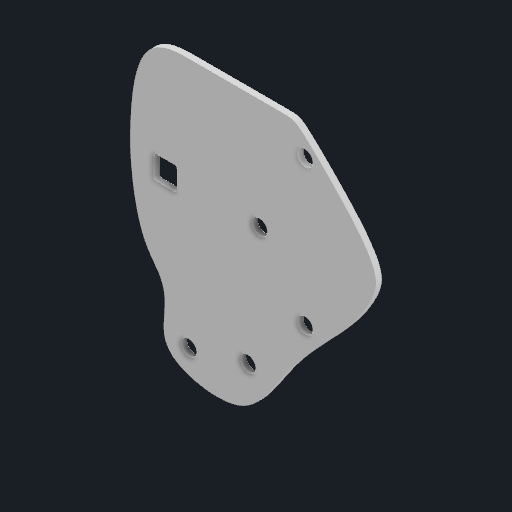
# Autodesk Inventor part: tracking-wheet-outer-mount-v2
Saved by Autodesk Inventor 2023.2 (Build 272271000, 271)
## iProperties
Created: 2023-04-12
Part Number: tracking-wheet-outer-mount-v2
Material: Generic
Document SubType Name: Modeling
Designer: Liam
Density: 1 g/cm^3
Appearance: Default
Author: Liam
Autodesk Inventor part; units mm, degrees
ref_plane "YZ Plane" through (0, 0, 0) normal (1, 0, 0) x (0, 1, 0)
ref_plane "XZ Plane" through (0, 0, 0) normal (0, 1, 0) x (-1, 0, 0)
ref_plane "XY Plane" through (0, 0, 0) normal (0, 0, 1) x (1, 0, 0)
sketch "Sketch1" plane through (0, 0, 0) normal (0, 0, 1) x (1, 0, 0)
  circle A0 centre (13.9823, 30.134) radius 2.0955 projected
  circle A1 centre (13.9823, -8.8165) radius 2.0955 projected
  circle A2 centre (-1.3811, -25.4474) radius 2.0955 projected
  circle A3 centre (-17.2724, -29.6635) radius 2.0955 projected
  line L0 (-20.518, 10.4175) -> (-20.518, 5.3883)
  line L1 (-21.153, 4.7533) -> (-26.1822, 4.7533)
  line L2 (-26.8172, 5.3883) -> (-26.8172, 10.4175)
  line L3 (-26.1822, 11.0525) -> (-21.153, 11.0525)
  arc A4 (-20.518, 10.4175) -> (-21.153, 11.0525) centre (-21.153, 10.4175) ccw
  arc A5 (-21.153, 4.7533) -> (-20.518, 5.3883) centre (-21.153, 5.3883) ccw
  arc A6 (-26.8172, 5.3883) -> (-26.1822, 4.7533) centre (-26.1822, 5.3883) ccw
  arc A7 (-26.1822, 11.0525) -> (-26.8172, 10.4175) centre (-26.1822, 10.4175) ccw
  line L4 (-23.6676, 7.9029) -> (-23.6676, 4.7533) construction
  line L5 (-23.6676, 7.9029) -> (-20.518, 7.9029) construction
  circle A8 centre (1.7324, 7.9029) radius 2.0955
  spline S0 degree 4 poles (-33.0614, 10.6587) (-33.0614, 4.3619) (-30.7457, -10.912) (-26.1565, -14.0262) (-21.9406, -21.3181) (-26.8507, -33.1) (-14.4545, -37.7063) (-3.2273, -37.7063) (3.1129, -31.759) (9.04, -21.3181) (16.0778, -13.5219) (22.0281, -7.3551) (28.8094, -0.0648) (33.0614, 7.9099) (33.0614, 10.6587) knots -12 -12 -12 -12 -12 -11 -10 -9 -8 -7 -6 -5 -4 -3 -2 -1 -1 -1 -1 -1 projected
  spline S1 degree 4 poles (33.0614, 10.6587) (33.0614, 15.0888) (24.5573, 25.0103) (12.2936, 37.1336) (10.8364, 37.7063) (6.7243, 37.7063) (3.0914, 37.7063) (-3.2273, 37.7063) (-7.0886, 37.7063) (-21.8204, 37.7063) (-24.0886, 37.7063) (-33.0614, 31.906) (-33.0614, 10.6587) knots -10 -10 -10 -10 -10 -9 -8 -7 -6 -5 -4 -3 -2 -1 -1 -1 -1 -1 projected
  point P0 (0, 0)
  point P1 (-20.518, 11.0525)
  point P2 (-20.518, 4.7533)
  dimension "d0" = 6.2992
  dimension "d1" = 0.635
  dimension "d2" = 3.1496
  dimension "d3" = 3.1496
  dimension "d4" = 4.191
  dimension "d5" = 0
  dimension "d6" = 25.4
  constraints: 12 end point, 8 point on circle, 8 tangent, 5 centre point, 4 point on line, 3 equal radius, 3 perpendicular, 2 midpoint, 1 horizontal, 1 vertical, 1 other
  measures "d0" distance of point (-20.518, 11.052) point (-20.518, 4.753)
  measures "d1" radius of A4
  measures "d2" distance of L4.start L5.end
  measures "d3" distance of L4.start L4.end
  measures "d4" diameter of A8
  measures "d5" vertical distance of L4.start A8.centre
  measures "d6" distance of L4.start A8.centre
extrude "Extrusion1" add sketch "Sketch1" along normal blind 1.524
equation "\"d2\" = 0.5 * d0"
equation "\"d3\" = d2"
body "Solid1"
